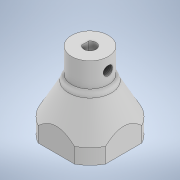
# Autodesk Inventor part: MocowanieChwytakaElement1
Saved by Autodesk Inventor 2021 (Build 250183000, 183)
## iProperties
Created: 2021-05-05
Part Number: MocowanieChwytakaElement1
Material: Ogólny
Document SubType Name: Modeling
Designer: micha
Density: 1 g/cm^3
Appearance: Domyślna
Author: micha
Autodesk Inventor part; units mm, degrees
ref_plane "YZ Plane" through (0, 0, 0) normal (1, 0, 0) x (0, 1, 0)
ref_plane "XZ Plane" through (0, 0, 0) normal (0, 1, 0) x (-1, 0, 0)
ref_plane "XY Plane" through (0, 0, 0) normal (0, 0, 1) x (1, 0, 0)
sketch "Szkic2" plane through (0, 0, 0) normal (0, 1, 0) x (-1, 0, 0)
  line L0 (-6, 6) -> (6, 6)
  line L1 (6, 6) -> (6, -6)
  line L2 (6, -6) -> (-6, -6)
  line L3 (-6, -6) -> (-6, 6)
  line L4 (-6, 6) -> (6, -6) construction
  line L5 (6, 6) -> (-6, -6) construction
  point P0 (0, 0)
  dimension "d3" = 12
  dimension "d4" = 12
  constraints: 12 end point, 2 midpoint, 2 parallel, 1 horizontal, 1 perpendicular
  measures "d3" distance of L1.end L2.end
  measures "d4" distance of L0.end L1.end
extrude "Wyciągnięcie proste1" add sketch "Szkic2" along normal blind 8
sketch "Szkic5" plane through (-6, 0, -6) normal (-1, 0, 0) x (0, 0, 1)
  line L0 (0, 8) -> (12, 8) projected
  line L1 (6, 8) -> (6, 0)
  line L2 (6, 0) -> (6, 8)
  line L3 (6, 8) -> (6, 4)
  circle A0 centre (6, 4) radius 1.5
  dimension "d10" = 4
  dimension "d11" = 3
  constraints: 6 end point, 2 midpoint, 1 centre point, 1 coincident, 1 collinear, 1 vertical
  measures "d10" distance of L1.start L3.end
  measures "d11" diameter of A0
extrude "Wyciągnięcie proste2" cut sketch "Szkic5" against normal through all
thread "Gwint1" size "M3x0.5" class "6H" standard "ANSI Metric M Profile" full length
sketch "Szkic6" plane through (0, 0, 0) normal (0, -1, 0) x (1, 0, 0)
  circle A0 centre (0, 0) radius 6
  circle A1 centre (0, 0) radius 8
  circle A2 centre (0, 0) radius 2
  line L0 (0, 0) -> (2, 0)
  line L1 (0, 0) -> (-1.6, 0)
  line L2 (-1.6, 0) -> (-1.6, -1.2)
  line L3 (-1.6, 0) -> (-1.6, 1.2)
  line L4 (-6, 6) -> (6, 6) projected
  circle A3 centre (0, 0) radius 8.4853
  point P0 (-5.2915, 6)
  point P1 (5.2915, 6)
  point P2 (0, 6)
  constraints: 8 end point, 4 coincident, 3 centre point, 3 point on circle, 2 horizontal, 1 perpendicular, 1 vertical, 3 other
extrude "Wyciągnięcie proste3" cut sketch "Szkic6" against normal blind 8 contours L4 A1 | L4 A3 A1 | A1 L4 A3 | L0 L1 L3 A2 | A2 L2 L1 L0 picked at (7.1897, -1.149)
sketch "Szkic11" plane through (0, 0, 0) normal (0, -1, 0) x (1, 0, 0)
  circle A0 centre (0, 0) radius 6
  circle A1 centre (0, 0) radius 7
  dimension "d24" = 14
  constraints: 2 centre point, 2 coincident
  measures "d24" diameter of A1
extrude "Wyciągnięcie proste4" add sketch "Szkic11" along normal blind 12 contours A0 | A1
sketch "Szkic18" plane through (0, -12, 0) normal (0, -1, 0) x (1, 0, 0)
  arc A0 (-1.6, -1.2) -> (-1.6, 1.2) centre (0, 0) ccw projected
  circle A1 centre (0, 0) radius 12.5
  dimension "d35" = 25
  constraints: 1 centre point, 1 coincident
  measures "d35" diameter of A1
loft "Wyciągnięcie złożone2" add profiles "Szkic18" section 2 edges at (0, 0, -6)
sketch "Szkic19" plane through (0, -12, 0) normal (0, -1, 0) x (1, 0, 0)
  circle A0 centre (0, 0) radius 12.5
  constraints: 1 centre point, 1 coincident
sketch "Szkic20" plane through (0, -12, 0) normal (0, -1, 0) x (1, 0, 0)
  point P0 (0, 0)
extrude "Wyciągnięcie proste6" add sketch "Szkic19" along normal blind 5
sketch "Szkic21" plane through (0, -17, 0) normal (0, -1, 0) x (1, 0, 0)
  line L0 (-11, 11) -> (11, 11)
  line L1 (11, 11) -> (11, -11)
  line L2 (11, -11) -> (-11, -11)
  line L3 (-11, -11) -> (-11, 11)
  circle A0 centre (0, 0) radius 6 projected
  line L4 (-11, 11) -> (11, -11) construction
  line L5 (11, 11) -> (-11, -11) construction
  circle A1 centre (0, 0) radius 12.5
  point P0 (5.9372, 11)
  point P1 (-5.9372, 11)
  point P2 (11, 5.9372)
  point P3 (11, -5.9372)
  point P4 (-11, 5.9372)
  point P5 (-11, -5.9372)
  point P6 (-5.9372, -11)
  point P7 (5.9372, -11)
  dimension "d42" = 22
  dimension "d43" = 22
  constraints: 12 end point, 2 midpoint, 2 parallel, 1 centre point, 1 coincident, 1 horizontal, 1 perpendicular
  measures "d42" distance of L1.end L2.end
  measures "d43" distance of L0.end L1.end
extrude "Wyciągnięcie proste7" cut sketch "Szkic21" against normal through all contours A1 L0 | L3 A1 | A1 L1 | L2 A1
sketch "Szkic22" plane through (0, -17, 0) normal (0, -1, 0) x (1, 0, 0)
  line L0 (0, 0) -> (-7, 0)
  line L1 (0, 0) -> (7, 0)
  circle A0 centre (-7, 0) radius 1.5
  circle A1 centre (7, 0) radius 1.5
  dimension "d46" = 7
  dimension "d47" = 7
  dimension "d48" = 3
  dimension "d49" = 3
  constraints: 4 end point, 2 centre point, 2 coincident, 2 horizontal
  measures "d46" distance of L0.start L0.end
  measures "d47" distance of L0.start L1.end
  measures "d48" diameter of A0
  measures "d49" diameter of A1
extrude "Wyciągnięcie proste8" cut sketch "Szkic22" against normal blind 5
thread "Gwint2" size "M3x0.5" class "6H" standard "ANSI Metric M Profile" full length
thread "Gwint3" size "M3x0.5" class "6H" standard "ANSI Metric M Profile" full length
fillet "Zaokrąglenie1" radius 2.2 1 edges at (-7, 0, 0)
